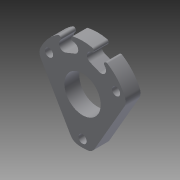
# Autodesk Inventor part: LowerPlate
Saved by Autodesk Inventor 2014 SP1 (Build 180222100, 222)
## iProperties
Created: 2013-12-26
Part Number: LowerPlate
Material: Generic
Document SubType Name: Modeling
Designer: Jack
Density: 1 g/cm^3
Appearance: Default
Author: Jack
Autodesk Inventor part; units mm, degrees
ref_plane "YZ Plane" through (0, 0, 0) normal (1, 0, 0) x (0, 1, 0)
ref_plane "XZ Plane" through (0, 0, 0) normal (0, 1, 0) x (-1, 0, 0)
ref_plane "XY Plane" through (0, 0, 0) normal (0, 0, 1) x (1, 0, 0)
sketch "Sketch1" plane through (0, 0, 0) normal (0, 1, 0) x (-1, 0, 0)
  circle A0 centre (-0.0038, -16.5528) radius 1.75
  circle A1 centre (-0.0038, -0.0528) radius 7.75
  circle A2 centre (-14.2932, 8.1972) radius 1.75
  circle A3 centre (14.2856, 8.1972) radius 1.75
  arc A4 (3.9019, 17.421) -> (3.1441, 13.3853) centre (3.9353, 15.3257) ccw
  arc A5 (3.9019, 17.421) -> (4.0803, 19.2703) centre (3.8869, 18.3557) ccw
  arc A6 (4.0803, 19.2703) -> (-4.0878, 19.2703) centre (-0.0038, -0.0528) ccw
  arc A7 (-4.0878, 19.2703) -> (-3.9094, 17.421) centre (-3.8945, 18.3557) ccw
  arc A8 (-3.1517, 13.3853) -> (-3.9094, 17.421) centre (-3.9429, 15.3257) ccw
  line L0 (-3.1517, 13.3853) -> (-7.1501, 11.755)
  arc A9 (-9.4303, 15.1698) -> (-7.1501, 11.755) centre (-7.9413, 13.6954) ccw
  arc A10 (-9.4303, 15.1698) -> (-10.596, 16.6166) centre (-10.0946, 15.8276) ccw
  arc A11 (-10.596, 16.6166) -> (-18.0415, 7.991) centre (-0.0038, -0.0528) ccw
  arc A12 (-18.0415, 7.991) -> (-17.8524, 4.3619) centre (-14.3883, 6.3619) ccw
  line L1 (-17.8524, 4.3619) -> (-5.1048, -17.7175)
  arc A13 (-5.1048, -17.7175) -> (-2.0565, -19.6958) centre (-1.6407, -15.7175) ccw
  arc A14 (-2.0565, -19.6958) -> (2.0489, -19.6958) centre (-0.0038, -0.0528) ccw
  arc A15 (2.0489, -19.6958) -> (5.0973, -17.7175) centre (1.6332, -15.7175) ccw
  line L2 (5.0973, -17.7175) -> (17.8448, 4.3619)
  arc A16 (17.8448, 4.3619) -> (18.0339, 7.991) centre (14.3807, 6.3619) ccw
  arc A17 (18.0339, 7.991) -> (10.5884, 16.6166) centre (-0.0038, -0.0528) ccw
  arc A18 (10.5884, 16.6166) -> (9.4227, 15.1698) centre (10.087, 15.8276) ccw
  arc A19 (7.1425, 11.755) -> (9.4227, 15.1698) centre (7.9337, 13.6954) ccw
  line L3 (7.1425, 11.755) -> (3.1441, 13.3853)
  constraints: 32 point on circle, 20 centre point, 8 end point
extrude "Extrusion1" add sketch "Sketch1" along normal blind 6.35
body "Solid1"
